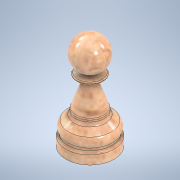
# Autodesk Inventor part: pionek
Saved by Autodesk Inventor 2021 (Build 250183000, 183)
## iProperties
Created: 2021-01-07
Part Number: pionek
Material: Drewno (brzoza)
Document SubType Name: Modeling
Designer: Adam
Density: 0.55 g/cm^3
Appearance: Brzoza — naturalna — polerowana
Author: Adam
Autodesk Inventor part; units mm, degrees
ref_plane "YZ Plane" through (0, 0, 0) normal (1, 0, 0) x (0, 1, 0)
ref_plane "XZ Plane" through (0, 0, 0) normal (0, 1, 0) x (-1, 0, 0)
ref_plane "XY Plane" through (0, 0, 0) normal (0, 0, 1) x (1, 0, 0)
sketch "Szkic1" plane through (0, 0, 0) normal (1, 0, 0) x (0, 1, 0)
  line L0 (20, -6) -> (20, -17)
  line L1 (20, -6) -> (64, -6)
  line L2 (20, -17) -> (25, -17)
  line L3 (25, -17) -> (25, -16)
  line L4 (25, -16) -> (26, -16)
  line L5 (26, -16) -> (26, -17)
  line L6 (26, -17) -> (29, -17)
  line L7 (29, -6) -> (33, -6)
  line L8 (29, -17) -> (33, -12.5279)
  line L9 (33, -12.5279) -> (35, -12.5279)
  line L10 (35, -6) -> (48, -6)
  line L11 (48, -8) -> (35, -12.5279)
  line L12 (48, -8) -> (48, -12)
  line L13 (48, -12) -> (49, -12)
  line L14 (49, -12) -> (50, -8)
  arc A0 (49.9037, -8.3854) -> (64, -6) centre (56.75, -6) ccw
  point P0 (0, 0)
  constraints: 30 end point, 8 point on line, 3 horizontal, 3 perpendicular, 2 point on circle, 2 vertical, 1 centre point
revolve "Obrót1" add sketch "Szkic1" angle 360 about axis through (0, 20, -6) along (0, 1, 0)
fillet "Zaokrąglenie1" radius 1 1 edges at (0, 25, 5)
fillet "Zaokrąglenie2" radius 3 2 edges at (0, 26, 5) (0, 29, 5)
fillet "Zaokrąglenie3" radius 0.5 2 edges at (0, 49, 0) (0, 48, 0)
fillet "Zaokrąglenie4" radius 2 2 edges at (0, 35, 0.5279) (0, 33, 0.5279)
